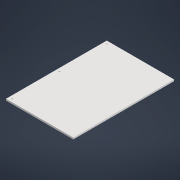
# Autodesk Inventor part: slide_panel
Saved by Autodesk Inventor 2021 (Build 250183000, 183)
## iProperties
Created: 2023-03-30
Part Number: slide_panel
Material: 木材(サクラ)
Document SubType Name: Modeling
Designer: casey
Density: 0.63 g/cm^3
Appearance: サクラ材 - ナチュラル 抑えた光沢
Author: casey
Autodesk Inventor part; units mm, degrees
ref_plane "YZ Plane" through (0, 0, 0) normal (1, 0, 0) x (0, 1, 0)
ref_plane "XZ Plane" through (0, 0, 0) normal (0, 1, 0) x (-1, 0, 0)
ref_plane "XY Plane" through (0, 0, 0) normal (0, 0, 1) x (1, 0, 0)
sketch "スケッチ1" plane through (0, 0, 0) normal (0, 1, 0) x (-1, 0, 0)
  line L0 (0, 0) -> (155, 0)
  line L1 (155, 0) -> (155, -240)
  line L2 (155, -240) -> (0, -240)
  line L3 (0, -240) -> (0, 0)
  dimension "d0" = 155
  dimension "d1" = 240
  constraints: 8 end point, 2 parallel, 1 horizontal, 1 perpendicular
  measures "d0" distance of L1.end L2.end
  measures "d1" distance of L0.end L1.end
extrude "押し出し1" add sketch "スケッチ1" along normal blind 4
sketch "スケッチ3" plane through (0, 4, 0) normal (0, 1, 0) x (1, 0, 0)
  line L0 (-155, 240) -> (-155, 0) projected
  line L1 (-155, 0) -> (0, 0) projected
  line L2 (0, 240) -> (-155, 240) projected
  point P0 (-150, 5)
  point P1 (-150, 235)
  point P2 (-150, 120)
  point P3 (-155, 120)
  dimension "d11" = 5
  dimension "d12" = 5
  dimension "d13" = 5
  dimension "d14" = 5
  dimension "d15" = 5
  dimension "d16" = 0
  constraints: 1 midpoint
  measures "d11" distance from line of L0 point (-150, 5)
  measures "d12" distance from line of point (-150, 5) L1
  measures "d13" distance from line of L0 point (-150, 235)
  measures "d14" distance from line of point (-150, 235) L2
  measures "d15" distance from line of L0 point (-150, 120)
  measures "d16" vertical distance of point (-150, 120) point (-155, 120)
hole "穴1" at (-150, 4, -5) at (-150, 4, -235) at (-150, 4, -120) direction (0, -1, 0) diameter 3.5 end through all
sketch "スケッチ5" plane through (0, 0, 0) normal (0, -1, 0) x (1, 0, 0)
  line L0 (0, -90) -> (0, -150) construction
  line L1 (0, 0) -> (0, -240) projected
  line L2 (-40, -90) -> (-40, -150)
  line L3 (40, -150) -> (40, -90)
  arc A0 (40, -90) -> (-40, -90) centre (0, -90) ccw
  arc A1 (-40, -150) -> (40, -150) centre (0, -150) ccw
  point P0 (0, -120)
  point P1 (0, -190)
  point P2 (0, -50)
  dimension "d17" = 80
  dimension "d18" = 30
  constraints: 8 end point, 4 point on circle, 4 tangent, 2 centre point, 2 midpoint, 1 parallel, 1 point on line
  measures "d17" diameter of A1
  measures "d18" distance of point (0, -120) L0.end
extrude "押し出し2" cut sketch "スケッチ5" against normal blind 10 contours L1 A1 L2 A0
sketch "スケッチ6" plane through (0, 0, 0) normal (0, -1, 0) x (1, 0, 0)
  line L0 (0, -240) -> (-155, -240) projected
  line L1 (0, -190) -> (0, -240) projected
  line L2 (-155, 0) -> (0, 0) projected
  line L3 (0, 0) -> (0, -50) projected
  point P0 (-20, -235)
  point P1 (-140, -235)
  point P2 (-140, -5)
  point P3 (-20, -5)
  dimension "d28" = 120
  dimension "d30" = 20
  dimension "d31" = 5
  dimension "d32" = 5
  dimension "d33" = 120
  dimension "d34" = 5
  dimension "d35" = 20
  dimension "d36" = 5
  measures "d28" distance of point (-20, -235) point (-140, -235)
  measures "d30" distance from line of L1 point (-20, -235)
  measures "d31" distance from line of L0 point (-20, -235)
  measures "d32" distance from line of L0 point (-140, -235)
  measures "d33" distance of point (-140, -5) point (-20, -5)
  measures "d34" distance from line of L2 point (-20, -5)
  measures "d35" distance from line of L3 point (-20, -5)
  measures "d36" distance from line of L2 point (-140, -5)
hole "穴2" at (-20, 0, -235) at (-140, 0, -235) at (-140, 0, -5) at (-20, 0, -5) direction (0, 1, 0) diameter 3.5 end through all
fillet "フィレット1" radius 10 2 edges at (0, 2, -50) (0, 2, -190)
